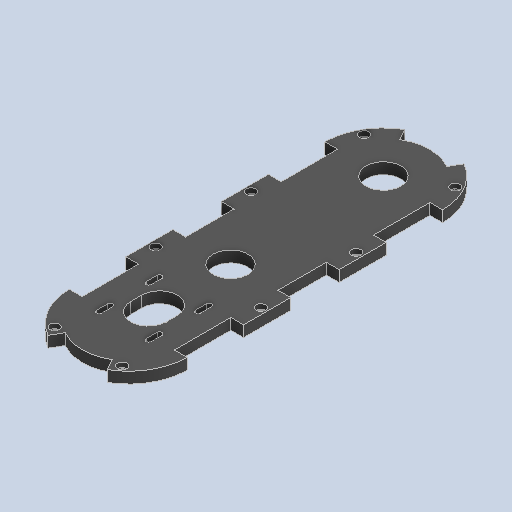
# Autodesk Inventor part: Segundo segmento - superior
Saved by Autodesk Inventor 2026 (Build 300175050, 175E)
## iProperties
Created: 2025-08-07
Part Number: Segundo segmento - superior
Material: Plastico PETG
Document SubType Name: Modeling
Designer: bello
Density: 1.27 g/cm^3
Appearance: Genérico
Author: bello
Autodesk Inventor part; units mm, degrees
ref_plane "YZ Plane" through (0, 0, 0) normal (1, 0, 0) x (0, 1, 0)
ref_plane "XZ Plane" through (0, 0, 0) normal (0, 1, 0) x (-1, 0, 0)
ref_plane "XY Plane" through (0, 0, 0) normal (0, 0, 1) x (1, 0, 0)
sketch "Boceto1" plane through (0, 0, 0) normal (0, 1, 0) x (-1, 0, 0)
  arc A0 (14.5, 25.1147) -> (0, 29) centre (0, 0) ccw
  arc A1 (0, -189) -> (14.5, -185.1147) centre (0, -160) ccw
  line L0 (37, 0) -> (29, 0)
  line L1 (37, -35) -> (29, -35)
  line L2 (29, -65) -> (37, -65)
  line L3 (29, -95) -> (37, -95)
  line L4 (29, -125) -> (37, -125)
  line L5 (29, -160) -> (37, -160)
  line L6 (14.5, 25.1147) -> (18.5, 32.0429)
  line L7 (14.5, -185.1147) -> (18.5, -192.0429)
  line L8 (0, 62.7565) -> (0, -215.9435)
  arc A2 (37, 0) -> (18.5, 32.0429) centre (0, 0) ccw
  line L9 (29, 0) -> (29, -35)
  line L10 (37, -35) -> (37, -65)
  line L11 (37, -95) -> (37, -125)
  line L12 (29, -65) -> (29, -95)
  line L13 (29, -125) -> (29, -160)
  arc A3 (18.5, -192.0429) -> (37, -160) centre (0, -160) ccw
  arc A4 (0, 29) -> (-14.5, 25.1147) centre (0, 0) ccw
  arc A5 (-14.5, -185.1147) -> (0, -189) centre (0, -160) ccw
  line L14 (-37, 0) -> (-29, 0)
  line L15 (-37, -35) -> (-29, -35)
  line L16 (-29, -65) -> (-37, -65)
  line L17 (-29, -95) -> (-37, -95)
  line L18 (-29, -125) -> (-37, -125)
  line L19 (-29, -160) -> (-37, -160)
  line L20 (-14.5, 25.1147) -> (-18.5, 32.0429)
  line L21 (-14.5, -185.1147) -> (-18.5, -192.0429)
  arc A6 (-18.5, 32.0429) -> (-37, 0) centre (0, 0) ccw
  line L22 (-29, 0) -> (-29, -35)
  line L23 (-37, -35) -> (-37, -65)
  line L24 (-37, -95) -> (-37, -125)
  line L25 (-29, -65) -> (-29, -95)
  line L26 (-29, -125) -> (-29, -160)
  arc A7 (-37, -160) -> (-18.5, -192.0429) centre (0, -160) ccw
  dimension "d1" = 58
  dimension "d3" = 58
  dimension "d4" = 160
  dimension "d5" = 35
  dimension "d6" = 30
  dimension "d7" = 30
  dimension "d8" = 30
  dimension "d9" = 35
  dimension "d10" = 60
  dimension "d11" = 60
  constraints: 54 end point, 16 point on circle, 16 symmetric about line, 14 perpendicular, 8 centre point, 5 coincident, 5 tangent, 2 point on line, 1 vertical, 4 other
  measures "d1" diameter of A0
  measures "d3" diameter of A1
  measures "d4" distance of A3.centre point (0, 0)
  measures "d5" distance between parallel lines of L0 L1
  measures "d6" distance between parallel lines of L1 L2
  measures "d7" distance between parallel lines of L2 L3
  measures "d8" distance between parallel lines of L4 L3
  measures "d9" distance between parallel lines of L4 L5
  measures "d10" angle of L6 L0
  measures "d11" angle of L5 L7
extrude "Extrusión1" add sketch "Boceto1" along normal blind 7
sketch "Boceto2" plane through (0, 7, 0) normal (0, 1, 0) x (1, 0, 0)
  circle A0 centre (-33, 50) radius 2.05
  circle A1 centre (-33, 110) radius 2.05
  arc A2 (-18.5, 192.0429) -> (-37, 160) centre (0, 160) ccw projected
  circle A3 centre (0, 160) radius 33
  circle A4 centre (0, 0) radius 33
  circle A5 centre (-21.212, -25.2795) radius 2.05
  line L0 (0, -60.8488) -> (0, 208.5153)
  circle A6 centre (-28.5788, 176.5) radius 2.05
  line L1 (-29, 65) -> (-37, 65) projected
  line L2 (-37, 65) -> (-37, 35) projected
  line L3 (-29, 125) -> (-37, 125) projected
  line L4 (-37, 125) -> (-37, 95) projected
  line L5 (-28.5788, 176.5) -> (0, 160)
  line L6 (0, 0) -> (-21.212, -25.2795)
  line L7 (-29, 0) -> (-37, 0) projected
  line L8 (-37, 160) -> (-29, 160) projected
  circle A7 centre (33, 50) radius 2.05
  circle A8 centre (33, 110) radius 2.05
  circle A9 centre (21.212, -25.2795) radius 2.05
  circle A10 centre (28.5788, 176.5) radius 2.05
  dimension "d14" = 66
  dimension "d15" = 66
  dimension "d16" = 4.1
  dimension "d17" = 15
  dimension "d18" = 4
  dimension "d19" = 15
  dimension "d20" = 4
  dimension "d21" = 50
  dimension "d22" = 30
  constraints: 8 centre point, 6 end point, 4 symmetric about line, 3 equal radius, 2 coincident, 1 vertical, 10 other
  measures "d16" diameter of A0
  measures "d17" distance from line of L1 A0.centre
  measures "d18" distance from line of L2 A0.centre
  measures "d19" distance from line of A1.centre L3
  measures "d20" distance from line of L4 A1.centre
  measures "d21" angle of L6 L7
  measures "d22" angle of L8 L5
extrude "Extrusión2" cut sketch "Boceto2" against normal through all contours A0 | A1 | A10 A3 | A3 A10 | A6 A3 | A3 L5 A6 | L5 A3 A6 | A9 A4 | A4 A9 | A5 L6 A4 | A4 A5 | A5 A4 L6 | A7 | A8
sketch "Boceto3" plane through (0, 7, 0) normal (0, 1, 0) x (1, 0, 0)
  circle A0 centre (-33, 50) radius 2.05 projected
  circle A1 centre (-33, 50) radius 3
  circle A2 centre (-33, 110) radius 2.05 projected
  circle A3 centre (-33, 110) radius 3
  circle A4 centre (-28.5788, 176.5) radius 2.05 projected
  circle A5 centre (-28.5788, 176.5) radius 3
  circle A6 centre (-21.212, -25.2795) radius 2.05 projected
  circle A7 centre (-21.212, -25.2795) radius 3
  line L0 (0, -43.6501) -> (0, 201.1209)
  circle A8 centre (33, 50) radius 2.05
  circle A9 centre (33, 50) radius 3
  circle A10 centre (33, 110) radius 2.05
  circle A11 centre (33, 110) radius 3
  circle A12 centre (28.5788, 176.5) radius 2.05
  circle A13 centre (28.5788, 176.5) radius 3
  circle A14 centre (21.212, -25.2795) radius 2.05
  circle A15 centre (21.212, -25.2795) radius 3
  point P0 (0, 0)
  dimension "d25" = 6
  constraints: 12 centre point, 8 coincident, 8 symmetric about line, 3 equal radius, 2 end point, 1 vertical, 8 other
  measures "d25" diameter of A1
extrude "Extrusión3" cut sketch "Boceto3" against normal blind 3 contours A0 | A1 | A2 | A3 | A4 | A5 | A6 | A7 | A8 | A9 | A10 | A11 | A12 | A13 | A14 | A15
sketch "Boceto4" plane through (0, 7, 0) normal (0, 1, 0) x (1, 0, 0)
  arc A0 (14.5, 185.1147) -> (-14.5, 185.1147) centre (0, 160) ccw projected
  arc A1 (-18.5, 192.0429) -> (-37, 160) centre (0, 160) ccw projected
  circle A2 centre (0, 160) radius 11
  circle A3 centre (0, 64) radius 11
  line L0 (0, 12.5) -> (0, 19.5) construction
  line L1 (11.1, 12.5) -> (11.1, 19.5)
  line L2 (-11.1, 19.5) -> (-11.1, 12.5)
  arc A4 (-11.1, 12.5) -> (11.1, 12.5) centre (0, 12.5) ccw
  arc A5 (11.1, 19.5) -> (-11.1, 19.5) centre (0, 19.5) ccw
  line L3 (-15.5, -3) -> (-15.5, 4) construction
  line L4 (-13.95, -3) -> (-13.95, 4)
  line L5 (-17.05, 4) -> (-17.05, -3)
  arc A6 (-17.05, -3) -> (-13.95, -3) centre (-15.5, -3) ccw
  arc A7 (-13.95, 4) -> (-17.05, 4) centre (-15.5, 4) ccw
  line L6 (4.1829, 16) -> (-3.8668, 16)
  line L7 (0, 6.9157) -> (0, 25.6477)
  line L8 (-15.5, 35) -> (-15.5, 28) construction
  line L9 (-13.95, 35) -> (-13.95, 28)
  line L10 (-17.05, 28) -> (-17.05, 35)
  arc A8 (-13.95, 35) -> (-17.05, 35) centre (-15.5, 35) ccw
  arc A9 (-17.05, 28) -> (-13.95, 28) centre (-15.5, 28) ccw
  line L11 (15.5, -3) -> (15.5, 4) construction
  line L12 (13.95, -3) -> (13.95, 4)
  line L13 (17.05, 4) -> (17.05, -3)
  arc A10 (13.95, -3) -> (17.05, -3) centre (15.5, -3) ccw
  arc A11 (17.05, 4) -> (13.95, 4) centre (15.5, 4) ccw
  arc A12 (13.95, 28) -> (17.05, 28) centre (15.5, 28) ccw
  line L14 (13.95, 35) -> (13.95, 28)
  line L15 (15.5, 35) -> (15.5, 28) construction
  arc A13 (17.05, 35) -> (13.95, 35) centre (15.5, 35) ccw
  line L16 (17.05, 28) -> (17.05, 35)
  point P0 (0, 189)
  point P1 (0, 16)
  point P2 (-15.5, 0.5)
  point P3 (-15.5, 31.5)
  point P4 (15.5, 0.5)
  point P5 (15.5, 31.5)
  dimension "d37" = 22
  dimension "d38" = 96
  dimension "d41" = 22.2
  dimension "d42" = 7
  dimension "d43" = 44.5
  dimension "d44" = 3.1
  dimension "d45" = 7
  dimension "d46" = 15.5
  dimension "d47" = 15.5
  constraints: 44 end point, 21 point on circle, 21 symmetric about line, 12 centre point, 8 tangent, 4 vertical, 2 midpoint, 2 parallel, 1 coincident, 1 equal radius, 1 horizontal, 6 other
  measures "d37" diameter of A2
  measures "d38" distance of A3.centre A0.centre
  measures "d41" distance between parallel lines of L1 L2
  measures "d42" distance of L2.start L2.end
  measures "d43" vertical distance of A3.centre L2.start
  measures "d44" distance between parallel lines of L4 L5
  measures "d45" distance of L5.start L5.end
  measures "d46" distance between parallel lines of L0 L3
  measures "d47" horizontal distance of L3.start L0.start
extrude "Extrusión4" cut sketch "Boceto4" against normal through all
sketch "Boceto7" plane through (0, 7, 0) normal (0, 1, 0) x (1, 0, 0)
  line L0 (-29, 65) -> (-37, 65) projected
  line L1 (-37, 65) -> (-29, 65)
  line L2 (-29, 65) -> (-29, 64.8)
  line L3 (-29, 64.8) -> (-37, 64.8)
  line L4 (-37, 64.8) -> (-37, 65)
  line L5 (-37, 35) -> (-29, 35) projected
  line L6 (-37, 35) -> (-29, 35)
  line L7 (-29, 35) -> (-29, 35.2)
  line L8 (-29, 35.2) -> (-37, 35.2)
  line L9 (-37, 35.2) -> (-37, 35)
  line L10 (-37, 125) -> (-37, 95) projected
  line L11 (-37, 95) -> (-29, 95)
  line L12 (-29, 95) -> (-29, 95.2)
  line L13 (-29, 95.2) -> (-37, 95.2)
  line L14 (-37, 95.2) -> (-37, 95)
  line L15 (-37, 125) -> (-29, 125)
  line L16 (-29, 125) -> (-29, 124.8)
  line L17 (-29, 124.8) -> (-37, 124.8)
  line L18 (-37, 124.8) -> (-37, 125)
  line L19 (-37, 160) -> (-29, 160) projected
  line L20 (-37, 160) -> (-29, 160)
  line L21 (-29, 160) -> (-29, 160.2)
  line L22 (-29, 160.2) -> (-37, 160.2)
  line L23 (-37, 160.2) -> (-37, 160)
  line L24 (-29, 0) -> (-37, 0) projected
  line L25 (-37, 0) -> (-29, 0)
  line L26 (-29, 0) -> (-29, -0.2)
  line L27 (-29, -0.2) -> (-37, -0.2)
  line L28 (-37, -0.2) -> (-37, 0)
  line L29 (-14.5, 185.1147) -> (-18.5, 192.0429) projected
  line L30 (-14.5, 185.1147) -> (-14.6732, 185.0147)
  line L31 (-14.6732, 185.0147) -> (-18.6732, 191.9429)
  arc A0 (-18.5, 192.0429) -> (-37, 160) centre (0, 160) ccw projected
  line L32 (-18.6732, 191.9429) -> (-18.5, 192.0429)
  line L33 (-18.5, -32.0429) -> (-14.5, -25.1147) projected
  line L34 (-14.5, -25.1147) -> (-14.6732, -25.0147)
  line L35 (-14.6732, -25.0147) -> (-18.6732, -31.9429)
  arc A1 (-37, 0) -> (-18.5, -32.0429) centre (0, 0) ccw projected
  line L36 (-18.6732, -31.9429) -> (-18.5, -32.0429)
  line L37 (0, 208.262) -> (0, -50.4937)
  line L38 (29, 65) -> (37, 65)
  line L39 (37, 65) -> (29, 65)
  line L40 (29, 65) -> (29, 64.8)
  line L41 (29, 64.8) -> (37, 64.8)
  line L42 (37, 64.8) -> (37, 65)
  line L43 (37, 35) -> (29, 35)
  line L44 (37, 35) -> (29, 35)
  line L45 (29, 35) -> (29, 35.2)
  line L46 (29, 35.2) -> (37, 35.2)
  line L47 (37, 35.2) -> (37, 35)
  line L48 (37, 125) -> (37, 95)
  line L49 (37, 95) -> (29, 95)
  line L50 (29, 95) -> (29, 95.2)
  line L51 (29, 95.2) -> (37, 95.2)
  line L52 (37, 95.2) -> (37, 95)
  line L53 (37, 125) -> (29, 125)
  line L54 (29, 125) -> (29, 124.8)
  line L55 (29, 124.8) -> (37, 124.8)
  line L56 (37, 124.8) -> (37, 125)
  line L57 (37, 160) -> (29, 160)
  line L58 (37, 160) -> (29, 160)
  line L59 (29, 160) -> (29, 160.2)
  line L60 (29, 160.2) -> (37, 160.2)
  line L61 (37, 160.2) -> (37, 160)
  line L62 (29, 0) -> (37, 0)
  line L63 (37, 0) -> (29, 0)
  line L64 (29, 0) -> (29, -0.2)
  line L65 (29, -0.2) -> (37, -0.2)
  line L66 (37, -0.2) -> (37, 0)
  line L67 (14.5, 185.1147) -> (18.5, 192.0429)
  line L68 (14.5, 185.1147) -> (14.6732, 185.0147)
  line L69 (14.6732, 185.0147) -> (18.6732, 191.9429)
  arc A2 (37, 160) -> (18.5, 192.0429) centre (0, 160) ccw
  line L70 (18.6732, 191.9429) -> (18.5, 192.0429)
  line L71 (18.5, -32.0429) -> (14.5, -25.1147)
  line L72 (14.5, -25.1147) -> (14.6732, -25.0147)
  line L73 (14.6732, -25.0147) -> (18.6732, -31.9429)
  arc A3 (18.5, -32.0429) -> (37, 0) centre (0, 0) ccw
  line L74 (18.6732, -31.9429) -> (18.5, -32.0429)
  point P0 (-36.9995, -0.2)
  point P1 (-36.9995, 160.2)
  point P2 (-18.6729, 191.9425)
  point P3 (18.6729, 191.9425)
  point P4 (36.9995, 160.2)
  point P5 (36.9995, -0.2)
  point P6 (18.6729, -31.9425)
  dimension "d66" = 0.2
  constraints: 136 end point, 36 symmetric about line, 12 parallel, 11 perpendicular, 7 equal length, 6 horizontal, 6 point on line, 4 point on circle, 2 centre point, 2 tangent, 1 vertical, 2 other
  measures "d66" distance of L25.end L26.end
extrude "Extrusión7" cut sketch "Boceto7" against normal through all
